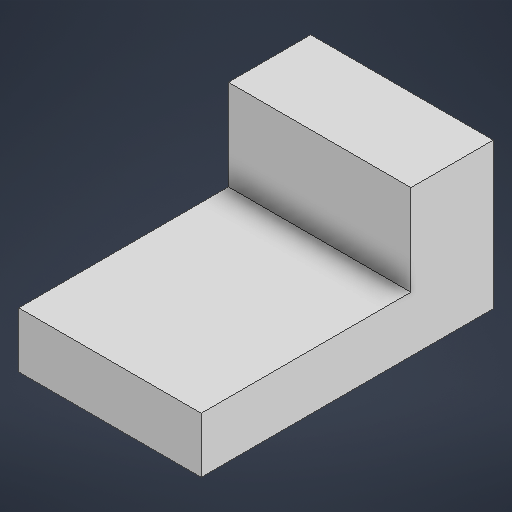
# Autodesk Inventor part: Peça_aula
Saved by Autodesk Inventor 2026 (Build 300175000, 175)
## iProperties
Created: 2026-03-13
Part Number: Peça_aula
Material: Genérico
Document SubType Name: Modeling
Designer: guisg
Density: 1 g/cm^3
Appearance: Padrão
Author: guisg
Autodesk Inventor part; units mm, degrees
ref_plane "YZ Plane" through (0, 0, 0) normal (1, 0, 0) x (0, 1, 0)
ref_plane "XZ Plane" through (0, 0, 0) normal (0, 1, 0) x (-1, 0, 0)
ref_plane "XY Plane" through (0, 0, 0) normal (0, 0, 1) x (1, 0, 0)
sketch "Esboço1" plane through (0, 0, 0) normal (1, 0, 0) x (0, 1, 0)
  line L0 (0, 0) -> (20, 0)
  line L1 (20, 0) -> (20, -40)
  line L2 (20, -40) -> (0, -40)
  line L3 (0, -40) -> (0, 0)
  dimension "d0" = 40
  dimension "d1" = 20
  constraints: 8 end point, 2 parallel, 1 horizontal, 1 perpendicular
  measures "d0" distance of L0.end L1.end
  measures "d1" distance of L1.end L2.end
extrude "Extrusão1" add sketch "Esboço1" along normal blind 25
sketch "Esboço2" plane through (25, 0, 0) normal (1, 0, 0) x (0, 0, -1)
  line L0 (28.7205, 20) -> (-11.2795, 20)
  line L1 (-11.2795, 20) -> (-11.2795, 7.5964)
  line L2 (-11.2795, 7.5964) -> (28.7205, 7.5964)
  line L3 (28.7205, 7.5964) -> (28.7205, 20)
  line L4 (0, 0) -> (40, 0) projected
  dimension "d4" = 40
  dimension "d5" = 20
  constraints: 8 end point, 2 parallel, 1 horizontal, 1 perpendicular
  measures "d4" distance of L0.start L0.end
  measures "d5" distance between parallel lines of L4 L0
extrude "Extrusão2" cut sketch "Esboço2" against normal through all
